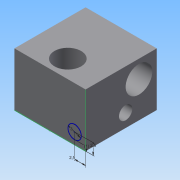
# Autodesk Inventor part: нагревательный  блок
Saved by Autodesk Inventor 2017 (Build 210142000, 142)
## iProperties
Part Number: нагревательный  блок
Material: Типовые
Document SubType Name: Modeling
Designer: Max
Mass: 2.28656 g
Surface Area: 24.185 cm^2
Volume: 2.28656 cm^3
Density: 1 g/cm^3
Appearance: Алюминий — темный
Author: Max
Autodesk Inventor part; units mm, degrees
ref_plane "YZ Plane" through (0, 0, 0) normal (1, 0, 0) x (0, 1, 0)
ref_plane "XZ Plane" through (0, 0, 0) normal (0, 1, 0) x (-1, 0, 0)
ref_plane "XY Plane" through (0, 0, 0) normal (0, 0, 1) x (1, 0, 0)
sketch "Эскиз1" plane through (0, 0, 0) normal (0, 0, 1) x (1, 0, 0)
  line L0 (8, 8) -> (-8, 8)
  line L1 (-8, 8) -> (-8, -8)
  line L2 (-8, -8) -> (8, -8)
  line L3 (8, -8) -> (8, 8)
  line L4 (8, 8) -> (-8, -8) construction
  line L5 (-8, 8) -> (8, -8) construction
  circle A0 centre (0, -4) radius 3
  circle A1 centre (0, 4) radius 1.5
  point P0 (0, 0)
  dimension "d0" = 16
  dimension "d1" = 16
  dimension "d2" = 6
  dimension "d3" = 3
  dimension "d4" = 4
  dimension "d5" = 4
  constraints: 12 end point, 2 centre point, 2 midpoint, 2 parallel, 1 horizontal, 1 perpendicular
  measures "d0" distance of L2.end L1.end
  measures "d1" distance of L1.end L0.end
  measures "d2" diameter of A0
  measures "d3" diameter of A1
  measures "d4" distance from line of A1.centre L0
  measures "d5" distance from line of L2 A0.centre
extrude "Выдавливание1" add sketch "Эскиз1" along normal blind 12 contours L3 L2 L1 L0 | A1
extrude "Выдавливание2" cut sketch "Эскиз1" along normal blind 1 contours A1
sketch "Эскиз2" plane through (8, -8, 0) normal (1, 0, 0) x (0, 0, -1)
  circle A0 centre (-8, 12) radius 3
  line L0 (0, 16) -> (-12, 16) projected
  line L1 (-12, 16) -> (-12, 0) projected
  circle A1 centre (-2.5, 9) radius 1.5
  line L2 (0, 0) -> (-12, 0) projected
  line L3 (0, 0) -> (0, 16) projected
  point P0 (0, 8)
  dimension "d10" = 6
  dimension "d11" = 4
  dimension "d12" = 4
  dimension "d13" = 3
  dimension "d14" = 9
  dimension "d15" = 2.5
  constraints: 2 centre point
  measures "d10" diameter of A0
  measures "d11" distance from line of L0 A0.centre
  measures "d12" distance from line of L1 A0.centre
  measures "d13" diameter of A1
  measures "d14" distance from line of L2 A1.centre
  measures "d15" distance from line of L3 A1.centre
extrude "Выдавливание3" cut sketch "Эскиз2" against normal blind 20 contours A0
extrude "Выдавливание4" cut sketch "Эскиз2" against normal blind 7 contours A1
sketch "Эскиз3" plane through (-8, -8, 0) normal (0, -1, 0) x (1, 0, 0)
  circle A0 centre (13.5, 2.5) radius 1.5
  line L0 (0, 0) -> (16, 0) projected
  line L1 (16, 0) -> (16, 12) projected
  point P0 (8, 0)
  dimension "d20" = 3
  dimension "d21" = 2.5
  dimension "d22" = 2.5
  dimension "d23" = 1
  constraints: 1 centre point
  measures "d20" diameter of A0
  measures "d21" distance from line of L0 A0.centre
  measures "d22" distance from line of A0.centre L1
  measures "d23" distance edge to line of A0 L0
extrude "Выдавливание5" cut sketch "Эскиз3" against normal blind 1
sketch "Эскиз4" plane through (5.5, -7, 2.5) normal (0, -1, 0) x (1, 0, 0)
  circle A0 centre (0, 0) radius 1.5 projected
  line L0 (0, -0.9132) -> (-0.7909, -0.4566)
  line L1 (-0.7909, -0.4566) -> (-0.7909, 0.4566)
  line L2 (-0.7909, 0.4566) -> (0, 0.9132)
  line L3 (0, 0.9132) -> (0.7909, 0.4566)
  line L4 (0.7909, 0.4566) -> (0.7909, -0.4566)
  line L5 (0.7909, -0.4566) -> (0, -0.9132)
  point P0 (-5.5, -2.5)
  constraints: 12 end point, 1 coincident, 13 other
extrude "Выдавливание6" cut sketch "Эскиз4" against normal blind 1 contours L0 L1 L2 L3 L4 L5
sketch "Эскиз5" plane through (0, 4, 1) normal (0, 0, -1) x (-1, 0, 0)
  line L0 (1.009, 0.0145) -> (0.517, -0.8666)
  line L1 (0.517, -0.8666) -> (-0.4919, -0.8811)
  line L2 (-0.4919, -0.8811) -> (-1.009, -0.0145)
  line L3 (-1.009, -0.0145) -> (-0.517, 0.8666)
  line L4 (-0.517, 0.8666) -> (0.4919, 0.8811)
  line L5 (0.4919, 0.8811) -> (1.009, 0.0145)
  point P0 (0, -4)
  point P1 (0, 0)
  constraints: 12 end point, 13 other
extrude "Выдавливание7" cut sketch "Эскиз5" against normal blind 1
thread "Резьба1" size "M3x0.5" class "6H" standard "ANSI Metric M Profile" full length
thread "Резьба2" size "M3x0.5" class "6H" standard "ANSI Metric M Profile" full length
sketch "Эскиз7" plane through (0, 4, 1) normal (-1, 0, 0) x (0, 1, 0)
  line L0 (1.5, 0) -> (1.5, 1)
  line L1 (1.5, 1) -> (1.1293, 1)
  line L2 (1.1293, 1) -> (1.1293, 0)
  line L3 (1.1293, 0) -> (1.5, 0)
  line L4 (0, -13.4) -> (0, 3.4) projected
  constraints: 8 end point
revolve "Вращение1" add sketch "Эскиз7" angle 360 about axis through (0, 4, 1) along (0, 0, -1) separate body
sketch "Эскиз6" plane through (0, 5.5, 1) normal (1, 0, 0) x (0, 0, -1)
  line L0 (-0.2918, -0.0255) -> (-0.2501, -0.0255) construction
  line L1 (0.0416, -0.3456) -> (-0.0001, -0.4257) construction
  line L2 (-0.5001, -0.4257) -> (-0.5418, -0.3456) construction
  line L3 (-0.2084, -0.0255) -> (-0.2501, 0.0546) construction
  line L4 (-0.2501, 0.0546) -> (-0.2918, -0.0255) construction
  line L5 (-0.5001, -0.4257) -> (-0.4584, -0.3456) construction
  line L6 (-0.2084, -0.0255) -> (-0.0418, -0.3456)
  line L7 (-0.5418, -0.3456) -> (-0.4584, -0.3456) construction
  arc A0 (-0.5418, -0.3456) -> (-0.5001, -0.3709) centre (-0.5001, -0.3239) ccw construction
  line L8 (0.0416, -0.3456) -> (-0.0418, -0.3456) construction
  line L9 (-0.5001, -0.4257) -> (-0.5001, -0.3456) construction
  line L10 (-0.0001, -0.4257) -> (-0.0001, -0.3456) construction
  line L11 (-0.2501, 0.0546) -> (-0.2501, -0.0002) construction
  line L12 (-0.5001, -0.3709) -> (-0.0001, -0.3709)
  arc A1 (-0.5001, -0.3709) -> (-0.4584, -0.3456) centre (-0.5001, -0.3239) ccw
  line L13 (-0.0418, -0.3456) -> (-0.0001, -0.4257) construction
  line L14 (-0.4584, -0.3456) -> (-0.2918, -0.0255)
  line L15 (-0.0001, -0.0002) -> (-0.0001, 0.0177)
  line L16 (-0.0001, 0.0177) -> (-0.0001, -0.0002)
  line L17 (-0.0001, -0.0002) -> (0.0334, -0.0002)
  arc A2 (-0.0418, -0.3456) -> (-0.0001, -0.3709) centre (-0.0001, -0.3239) ccw
  arc A3 (-0.0001, -0.3709) -> (0.0416, -0.3456) centre (-0.0001, -0.3239) ccw construction
  arc A4 (-0.2501, -0.0002) -> (-0.2918, -0.0255) centre (-0.2501, -0.0471) ccw
  arc A5 (-0.2084, -0.0255) -> (-0.2501, -0.0002) centre (-0.2501, -0.0471) ccw
  line L18 (-0.2501, -0.0002) -> (-0.2501, -0.0255) construction
  line L19 (-0.2501, -0.0255) -> (-0.2084, -0.0255) construction
  dimension "d34" = 55
  dimension "d35" = 0.08
  dimension "d36" = 0.08
  dimension "Эскиз6_ThreadOffset" = 0
  dimension "Эскиз6_MajorRadius" = 0.3707
  dimension "d39" = 0.5
  dimension "Эскиз6_MinorRadius" = 0
  constraints: 40 end point, 12 point on circle, 10 parallel, 8 tangent, 6 centre point, 6 collinear, 2 midpoint, 2 point on line, 1 horizontal, 1 perpendicular, 3 other
  measures "d34" angle of L6 L14
  measures "d35" distance of L3.end L0.end
  measures "d36" distance of L1.end L10.end
  measures "Эскиз6_ThreadOffset" distance between parallel lines of L15 L10
  measures "Эскиз6_MajorRadius" distance from line of L12 L15.start
  measures "d39" distance from line of L1.end L9
  measures "Эскиз6_MinorRadius" distance edge to line of A5 L17
coil "Пружина1" sketch "Эскиз6" operation cut axis through (0, 4, 1) along (0, 0, -1) pitch 0.5005 turns 3.996004 hand right bodies 2
sketch "Эскиз9" plane through (5.5, -7, 2.5) normal (1, 0, 0) x (0, 0, 1)
  line L0 (1.5, 0) -> (1.5, 1)
  line L1 (1.5, 1) -> (1.1293, 1)
  line L2 (1.1293, 1) -> (1.1293, 0)
  line L3 (1.1293, 0) -> (1.5, 0)
  line L4 (0, -18.2) -> (0, 4.2) projected
  constraints: 8 end point
revolve "Вращение2" add sketch "Эскиз9" angle 360 about axis through (5.5, -7, 2.5) along (0, -1, 0) separate body
sketch "Эскиз8" plane through (5.5, -7, 4) normal (-1, 0, 0) x (0, -1, 0)
  line L0 (-0.2918, -0.0255) -> (-0.2501, -0.0255) construction
  line L1 (0.0416, -0.3456) -> (-0.0001, -0.4257) construction
  line L2 (-0.5001, -0.4257) -> (-0.5418, -0.3456) construction
  line L3 (-0.2084, -0.0255) -> (-0.2501, 0.0546) construction
  line L4 (-0.2501, 0.0546) -> (-0.2918, -0.0255) construction
  line L5 (-0.5001, -0.4257) -> (-0.4584, -0.3456) construction
  line L6 (-0.2084, -0.0255) -> (-0.0418, -0.3456)
  line L7 (-0.5418, -0.3456) -> (-0.4584, -0.3456) construction
  arc A0 (-0.5418, -0.3456) -> (-0.5001, -0.3709) centre (-0.5001, -0.3239) ccw construction
  line L8 (0.0416, -0.3456) -> (-0.0418, -0.3456) construction
  line L9 (-0.5001, -0.4257) -> (-0.5001, -0.3456) construction
  line L10 (-0.0001, -0.4257) -> (-0.0001, -0.3456) construction
  line L11 (-0.2501, 0.0546) -> (-0.2501, -0.0002) construction
  line L12 (-0.5001, -0.3709) -> (-0.0001, -0.3709)
  arc A1 (-0.5001, -0.3709) -> (-0.4584, -0.3456) centre (-0.5001, -0.3239) ccw
  line L13 (-0.0418, -0.3456) -> (-0.0001, -0.4257) construction
  line L14 (-0.4584, -0.3456) -> (-0.2918, -0.0255)
  line L15 (-0.0001, -0.0002) -> (-0.0001, 0.0177)
  line L16 (-0.0001, 0.0177) -> (-0.0001, -0.0002)
  line L17 (-0.0001, -0.0002) -> (0.0334, -0.0002)
  arc A2 (-0.0418, -0.3456) -> (-0.0001, -0.3709) centre (-0.0001, -0.3239) ccw
  arc A3 (-0.0001, -0.3709) -> (0.0416, -0.3456) centre (-0.0001, -0.3239) ccw construction
  arc A4 (-0.2501, -0.0002) -> (-0.2918, -0.0255) centre (-0.2501, -0.0471) ccw
  arc A5 (-0.2084, -0.0255) -> (-0.2501, -0.0002) centre (-0.2501, -0.0471) ccw
  line L18 (-0.2501, -0.0002) -> (-0.2501, -0.0255) construction
  line L19 (-0.2501, -0.0255) -> (-0.2084, -0.0255) construction
  dimension "d52" = 55
  dimension "d53" = 0.08
  dimension "d54" = 0.08
  dimension "Эскиз8_ThreadOffset" = 0
  dimension "Эскиз8_MajorRadius" = 0.3707
  dimension "d57" = 0.5
  dimension "Эскиз8_MinorRadius" = 0
  constraints: 40 end point, 12 point on circle, 10 parallel, 8 tangent, 6 centre point, 6 collinear, 2 midpoint, 2 point on line, 1 horizontal, 1 perpendicular, 3 other
  measures "d52" angle of L6 L14
  measures "d53" distance of L3.end L0.end
  measures "d54" distance of L1.end L10.end
  measures "Эскиз8_ThreadOffset" distance between parallel lines of L15 L10
  measures "Эскиз8_MajorRadius" distance from line of L12 L15.start
  measures "d57" distance from line of L1.end L9
  measures "Эскиз8_MinorRadius" distance edge to line of A5 L17
coil "Пружина2" sketch "Эскиз8" operation cut axis through (5.5, -7, 2.5) along (0, -1, 0) pitch 0.5005 turns 3.996004 hand right bodies 3
fillet "Сопряжение1" radius 0.2 4 edges at (0, -8, 0) (0, 8, 0) (0, 8, 12) (0, -8, 12)
chamfer "Фаска1" distance 0.2 angle 45 5 edges at (8, 1, 4) (8, 4, 11) (-3, -4, 0) (-3, -4, 12) (-8, 4, 11)
thread "Резьба3" size "M6x1" class "6H" standard "ANSI Metric M Profile" full length
sketch "Эскиз11" plane through (0, -4, 11.8) normal (-1, 0, 0) x (0, 1, 0)
  line L0 (3, 0) -> (3, 11.6)
  line L1 (3, 11.6) -> (2.2585, 11.6)
  line L2 (2.2585, 11.6) -> (2.2585, 0)
  line L3 (2.2585, 0) -> (3, 0)
  line L4 (0, -3.7019) -> (0, 14.5781) projected
  constraints: 8 end point
revolve "Вращение3" add sketch "Эскиз11" angle 360 about axis through (0, -4, 11.8) along (0, 0, -1) separate body
sketch "Эскиз10" plane through (0, -1, 11.8) normal (1, 0, 0) x (0, 0, -1)
  line L0 (-0.5834, -0.0507) -> (-0.5001, -0.0507) construction
  line L1 (0.0832, -0.6911) -> (-0.0001, -0.8511) construction
  line L2 (-1.0001, -0.8511) -> (-1.0834, -0.6911) construction
  line L3 (-0.4168, -0.0507) -> (-0.5001, 0.1093) construction
  line L4 (-0.5001, 0.1093) -> (-0.5834, -0.0507) construction
  line L5 (-1.0001, -0.8511) -> (-0.9168, -0.6911) construction
  line L6 (-0.4168, -0.0507) -> (-0.0834, -0.6911)
  line L7 (-1.0834, -0.6911) -> (-0.9168, -0.6911) construction
  arc A0 (-1.0834, -0.6911) -> (-1.0001, -0.7416) centre (-1.0001, -0.6477) ccw construction
  line L8 (0.0832, -0.6911) -> (-0.0834, -0.6911) construction
  line L9 (-1.0001, -0.8511) -> (-1.0001, -0.6911) construction
  line L10 (-0.0001, -0.8511) -> (-0.0001, -0.6911) construction
  line L11 (-0.5001, 0.1093) -> (-0.5001, -0.0002) construction
  line L12 (-1.0001, -0.7416) -> (-0.0001, -0.7416)
  arc A1 (-1.0001, -0.7416) -> (-0.9168, -0.6911) centre (-1.0001, -0.6477) ccw
  line L13 (-0.0834, -0.6911) -> (-0.0001, -0.8511) construction
  line L14 (-0.9168, -0.6911) -> (-0.5834, -0.0507)
  line L15 (-0.0001, -0.0002) -> (-0.0001, 0.0177)
  line L16 (-0.0001, 0.0177) -> (-0.0001, -0.0002)
  line L17 (-0.0001, -0.0002) -> (0.0334, -0.0002)
  arc A2 (-0.0834, -0.6911) -> (-0.0001, -0.7416) centre (-0.0001, -0.6477) ccw
  arc A3 (-0.0001, -0.7416) -> (0.0832, -0.6911) centre (-0.0001, -0.6477) ccw construction
  arc A4 (-0.5001, -0.0002) -> (-0.5834, -0.0507) centre (-0.5001, -0.0941) ccw
  arc A5 (-0.4168, -0.0507) -> (-0.5001, -0.0002) centre (-0.5001, -0.0941) ccw
  line L18 (-0.5001, -0.0002) -> (-0.5001, -0.0507) construction
  line L19 (-0.5001, -0.0507) -> (-0.4168, -0.0507) construction
  dimension "d76" = 55
  dimension "d77" = 0.1601
  dimension "d78" = 0.1601
  dimension "Эскиз10_ThreadOffset" = 0
  dimension "Эскиз10_MajorRadius" = 0.7415
  dimension "d81" = 1
  dimension "Эскиз10_MinorRadius" = 0
  constraints: 40 end point, 12 point on circle, 10 parallel, 8 tangent, 6 centre point, 6 collinear, 2 midpoint, 2 point on line, 1 horizontal, 1 perpendicular, 3 other
  measures "d76" angle of L6 L14
  measures "d77" distance of L3.end L0.end
  measures "d78" distance of L1.end L10.end
  measures "Эскиз10_ThreadOffset" distance between parallel lines of L15 L10
  measures "Эскиз10_MajorRadius" distance from line of L12 L15.start
  measures "d81" distance from line of L1.end L9
  measures "Эскиз10_MinorRadius" distance edge to line of A5 L17
coil "Пружина3" sketch "Эскиз10" operation cut axis through (0, -4, 11.8) along (0, 0, -1) pitch 1.001 turns 13.586414 hand right bodies 4
equation "\"d34\" = d41"
equation "\"d35\" = 0.160083 * Эскиз6_Pitch"
equation "\"d36\" = 0.160083 * Эскиз6_Pitch"
equation "\"d39\" = Эскиз6_Pitch"
equation "\"d52\" = d59"
equation "\"d53\" = 0.160083 * Эскиз8_Pitch"
equation "\"d54\" = 0.160083 * Эскиз8_Pitch"
equation "\"d57\" = Эскиз8_Pitch"
equation "\"d76\" = d83"
equation "\"d77\" = 0.160083 * Эскиз10_Pitch"
equation "\"d78\" = 0.160083 * Эскиз10_Pitch"
equation "\"d81\" = Эскиз10_Pitch"
equation "\"d41\" = 55deg"
equation "\"Эскиз6_Pitch\" = 0.5"
equation "\"d59\" = 55deg"
equation "\"Эскиз8_Pitch\" = 0.5"
equation "\"d83\" = 55deg"
equation "\"Эскиз10_Pitch\" = 1"
